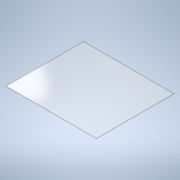
# Autodesk Inventor part: Electronics Lexan
Saved by Autodesk Inventor 2021 (Build 250183000, 183)
## iProperties
Created: 2020-01-14
Part Number: Electronics Lexan
Material: Polycarbonate, Clear
Document SubType Name: Modeling
Designer: aidan
Density: 1.2 g/cm^3
Appearance: Polycarbonate - Clear
Author: aidan
Autodesk Inventor part; units mm, degrees
ref_plane "YZ Plane" through (0, 0, 0) normal (1, 0, 0) x (0, 1, 0)
ref_plane "XZ Plane" through (0, 0, 0) normal (0, 1, 0) x (-1, 0, 0)
ref_plane "XY Plane" through (0, 0, 0) normal (0, 0, 1) x (1, 0, 0)
sketch "Sketch1" plane through (0, 0, 0) normal (0, 1, 0) x (-1, 0, 0)
  line L0 (374.9202, 269.9426) -> (-82.2798, 269.9426)
  line L1 (-82.2798, 269.9426) -> (-82.2798, -263.4574)
  line L2 (-82.2798, -263.4574) -> (374.9202, -263.4574)
  line L3 (374.9202, -263.4574) -> (374.9202, 269.9426)
  point P0 (0, 0)
  dimension "d0" = 533.4
  dimension "d1" = 457.2
  constraints: 8 end point, 2 parallel, 1 horizontal, 1 perpendicular
  measures "d0" distance of L2.end L0.start
  measures "d1" distance of L1.end L2.end
extrude "Extrusion1" add sketch "Sketch1" along normal blind 2.9972
body "Solid1"
